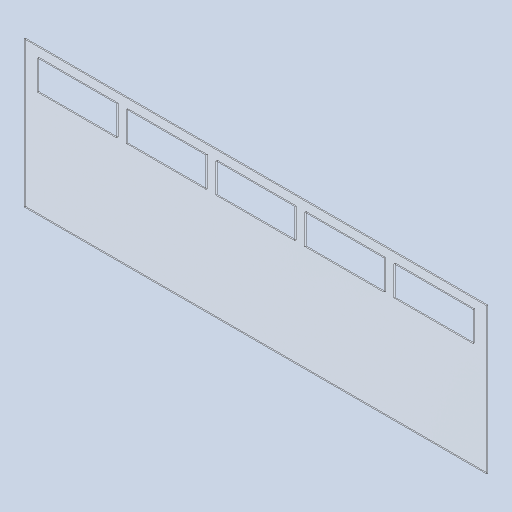
# Autodesk Inventor part: Lado
Saved by Autodesk Inventor 2025.1 (Build 291241000, 241)
## iProperties
Created: 2024-09-06
Part Number: Lado
Material: Acrylic
Document SubType Name: Modeling
Designer: joser
Density: 1.188 g/cm^3
Appearance: Transparent - Clear
Mass: 14434.2 g
Surface Area: 9885 cm^2
Volume: 12150 cm^3
Author: joser
Autodesk Inventor part; units mm, degrees
ref_plane "YZ Plane" through (0, 0, 0) normal (1, 0, 0) x (0, 1, 0)
ref_plane "XZ Plane" through (0, 0, 0) normal (0, 1, 0) x (-1, 0, 0)
ref_plane "XY Plane" through (0, 0, 0) normal (0, 0, 1) x (1, 0, 0)
sketch "Sketch1" plane through (0, 0, 0) normal (0, 0, 1) x (1, 0, 0)
  line L0 (-584, -184) -> (584, -184)
  line L1 (584, -184) -> (584, 184)
  line L2 (584, 184) -> (-584, 184)
  line L3 (-584, 184) -> (-584, -184)
  line L4 (-584, -184) -> (584, 184) construction
  line L5 (584, -184) -> (-584, 184) construction
  line L6 (-550, 159) -> (-350, 159)
  line L7 (-350, 159) -> (-350, 84)
  line L8 (-350, 84) -> (-550, 84)
  line L9 (-550, 84) -> (-550, 159)
  line L10 (-325, 84) -> (-325, 159)
  line L11 (-325, 159) -> (-125, 159)
  line L12 (-125, 159) -> (-125, 84)
  line L13 (-125, 84) -> (-325, 84)
  line L14 (-100, 84) -> (-100, 159)
  line L15 (-100, 159) -> (100, 159)
  line L16 (100, 159) -> (100, 84)
  line L17 (100, 84) -> (-100, 84)
  line L18 (125, 84) -> (125, 159)
  line L19 (125, 159) -> (325, 159)
  line L20 (325, 159) -> (325, 84)
  line L21 (325, 84) -> (125, 84)
  line L22 (350, 84) -> (350, 159)
  line L23 (350, 159) -> (550, 159)
  line L24 (550, 159) -> (550, 84)
  line L25 (550, 84) -> (350, 84)
  point P0 (0, 0)
  point P1 (-550, 121.5)
  point P2 (-325, 121.5)
  point P3 (-100, 121.5)
  point P4 (125, 121.5)
  point P5 (350, 121.5)
  dimension "d0" = 1168
  dimension "d1" = 368
  dimension "d2" = 75
  dimension "d3" = 25
  dimension "d4" = 200
  dimension "d5" = 34
  dimension "d10" = 225
  constraints: 52 end point, 4 parallel, 3 horizontal, 3 midpoint, 2 perpendicular, 36 other
  measures "d0" distance of L1.end L2.end
  measures "d1" distance of L0.end L1.end
  measures "d2" distance of L6.end L7.end
  measures "d3" vertical distance of L2.end L6.start
  measures "d4" distance of L7.end L8.end
  measures "d5" distance from line of L3 point (-550, 121.5)
  measures "d10" distance of L8.end L10.start
extrude "Extrusion2" add sketch "Sketch1" along normal mid plane 3
body "Solid2"
